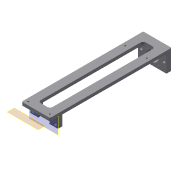
# Autodesk Inventor part: 02_Opentrons_Microscope_Base_v0
Saved by Autodesk Inventor 2019.4 (Build 234330000, 330)
## iProperties
Created: 2020-10-28
Part Number: 02_Opentrons_Microscope_Base_v0
Material: Generic
Document SubType Name: Modeling
Designer: diederichbenedict
Density: 1 g/cm^3
Appearance: Default
Author: diederichbenedict
Autodesk Inventor part; units mm, degrees
ref_plane "YZ Plane" through (0, 0, 0) normal (1, 0, 0) x (0, 1, 0)
ref_plane "XZ Plane" through (0, 0, 0) normal (0, 1, 0) x (-1, 0, 0)
ref_plane "XY Plane" through (0, 0, 0) normal (0, 0, 1) x (1, 0, 0)
ref_plane "Work Plane1" through (130.593, 54.6266, 280.0982) normal (0, 1, 0) x (1, 0, 0)
sketch "Sketch1" plane through (130.593, 54.6266, 280.0982) normal (0, 1, 0) x (1, 0, 0)
  line L0 (0, 36) -> (2, 38) projected
  line L1 (0, 27) -> (0, 36) projected
  line L2 (2, 25) -> (0, 27) projected
  line L3 (2, 25) -> (53, 25) projected
  line L4 (55, 27) -> (53, 25) projected
  line L5 (55, 27) -> (55, 36) projected
  line L6 (53, 38) -> (55, 36) projected
  line L7 (2, 38) -> (53, 38) projected
  circle A0 centre (6.5, 31.5) radius 2.5 construction
  circle A1 centre (48.5, 31.5) radius 2.5 construction
  line L8 (0, 224) -> (2, 226) projected
  line L9 (0, 215) -> (0, 224) projected
  line L10 (2, 213) -> (0, 215) projected
  line L11 (2, 213) -> (53, 213) projected
  line L12 (55, 215) -> (53, 213) projected
  line L13 (55, 215) -> (55, 224) projected
  line L14 (53, 226) -> (55, 224) projected
  line L15 (2, 226) -> (53, 226) projected
  circle A2 centre (6.5, 219.5) radius 2.5 construction
  circle A3 centre (48.5, 219.5) radius 2.5 construction
  line L16 (55, 25) -> (0, 25)
  line L17 (0, 25) -> (0, 261)
  line L18 (0, 261) -> (55, 261)
  line L19 (55, 261) -> (55, 25)
  line L20 (16, 261) -> (39, 261) projected
  circle A4 centre (48.5, 31.5) radius 1.45
  circle A5 centre (6.5, 31.5) radius 1.45
  circle A6 centre (48.5, 219.5) radius 1.45
  circle A7 centre (6.5, 219.5) radius 1.45
  point P0 (-130.593, 280.0982)
  dimension "d12" = 2.9
  dimension "d13" = 2.9
  dimension "d14" = 2.9
  dimension "d15" = 2.9
  constraints: 8 end point, 4 centre point, 3 coincident, 2 parallel, 2 point on line, 1 horizontal, 1 perpendicular
  measures "d12" diameter of A4
  measures "d13" diameter of A5
  measures "d14" diameter of A6
  measures "d15" diameter of A7
extrude "Extrusion1" add sketch "Sketch1" along normal blind 6
sketch "Sketch2" plane through (185.593, 54.6266, 19.0982) normal (0, 0, -1) x (-1, 0, 0)
  line L0 (46, 0) -> (46, 10) projected
  circle A0 centre (39, -26) radius 0.8 projected
  circle A1 centre (39, -3) radius 0.8 projected
  circle A2 centre (16, -26) radius 0.8 projected
  circle A3 centre (16, -3) radius 0.8 projected
  circle A4 centre (27.5, -14.5) radius 9.4 projected
  circle A5 centre (27.5, -14.5) radius 10.8 projected
  circle A6 centre (27.5, -14.5) radius 11.8
  circle A7 centre (5.5, -14.5) radius 3 projected
  circle A8 centre (49.5, -14.5) radius 3 projected
  circle A9 centre (5.5, -14.5) radius 3.1
  circle A10 centre (49.5, -14.5) radius 3.1
  line L1 (0, 0) -> (55, 0) projected
  line L2 (0, 0) -> (55, 0)
  line L3 (55, 0) -> (55, -32.5)
  line L4 (55, -32.5) -> (0, -32.5)
  line L5 (0, -32.5) -> (0, 0)
  point P0 (185.593, -54.6266)
  dimension "d2" = 1
  dimension "d3" = 6.2
  dimension "d4" = 6.2
  dimension "d5" = 18
  constraints: 8 end point, 3 centre point, 2 coincident, 2 parallel, 1 horizontal, 1 perpendicular
  measures "d2" radial gap between concentric circles of A5 A6
  measures "d3" diameter of A9
  measures "d4" diameter of A10
  measures "d5" distance from line of L4 A5.centre
extrude "Extrusion2" add sketch "Sketch2" against normal blind 10 contours L1 L3 L4 L5
ref_plane "Work Plane2" through (158.093, 40.1266, 239.5982) normal (0, 0, -1) x (1, 0, 0)
sketch "Sketch3" plane through (158.093, 40.1266, 239.5982) normal (0, 0, -1) x (1, 0, 0)
  circle A0 centre (-22, 0) radius 3 projected
  circle A1 centre (22, 0) radius 3 projected
  circle A2 centre (0, 0) radius 11.8 projected
  line L0 (27.5, -14.5) -> (27.5, -20.5) projected
  line L1 (-27.5, 18) -> (-27.5, -20.5) projected
  line L2 (27.5, -14.5) -> (-27.5, -14.5)
  line L3 (-27.5, -14.5) -> (-27.5, 5.5)
  line L4 (-27.5, 5.5) -> (27.5, 5.5)
  line L5 (27.5, 5.5) -> (27.5, -14.5)
  point P0 (-158.093, 40.1266)
  point P1 (10.4398, 5.5)
  point P2 (-10.4398, 5.5)
  dimension "d8" = 20
  constraints: 8 end point, 3 point on line, 2 parallel, 2 point on circle, 1 horizontal, 1 perpendicular
  measures "d8" distance of L2.end L3.end
extrude "Extrusion3" add sketch "Sketch3" along normal blind 10 contours A2 L4 L5 L2 L1
fillet "Fillet1" radius 2 9 edges at (185.593, 41.3766, 19.0982) (158.093, 54.6266, 29.0982) (185.593, 44.6266, 229.5982) (185.593, 44.6266, 239.5982) (130.593, 44.6266, 229.5982) (130.593, 44.6266, 239.5982) (130.593, 57.6266, 255.0982) (185.593, 57.6266, 255.0982) (130.593, 41.3766, 19.0982)
sketch "Sketch4" plane through (130.593, 60.6266, 280.0982) normal (0, 1, 0) x (1, 0, 0)
  arc A0 (2, 261) -> (0, 259) centre (2, 259) ccw construction
  line L0 (0, 259) -> (0, 27) construction
  arc A1 (0, 27) -> (2, 25) centre (2, 27) ccw construction
  line L1 (2, 25) -> (53, 25) construction
  arc A2 (53, 25) -> (55, 27) centre (53, 27) ccw construction
  line L2 (55, 27) -> (55, 259) construction
  arc A3 (55, 259) -> (53, 261) centre (53, 259) ccw construction
  line L3 (53, 261) -> (2, 261) construction
  circle A4 centre (6.5, 219.5) radius 1.45 projected
  circle A5 centre (48.5, 219.5) radius 1.45 projected
  circle A6 centre (6.5, 31.5) radius 1.45 projected
  circle A7 centre (48.5, 31.5) radius 1.45 projected
  line L4 (16, 46) -> (16, 240)
  line L5 (21, 245) -> (34, 245)
  line L6 (39, 240) -> (39, 46)
  line L7 (34, 41) -> (21, 41)
  arc A8 (16, 46) -> (21, 41) centre (21, 46) ccw
  arc A9 (34, 41) -> (39, 46) centre (34, 46) ccw
  arc A10 (39, 240) -> (34, 245) centre (34, 240) ccw
  arc A11 (21, 245) -> (16, 240) centre (21, 240) ccw
  point P0 (-130.593, 280.0982)
  dimension "d16" = 16
  dimension "d17" = 5
  constraints: 8 end point, 8 point on circle, 8 tangent, 4 centre point, 3 equal radius, 3 other
  measures "d16" distance between parallel lines of L0 L4
  measures "d17" radius of A8
extrude "Extrusion4" cut sketch "Sketch4" against normal through all contours L4 A11 L5 A10 L6 A9 L7 A8
sketch "Sketch5" plane through (130.593, 60.6266, 280.0982) normal (0, 1, 0) x (1, 0, 0)
  circle A0 centre (48.5, 219.5) radius 1.45 projected
  circle A1 centre (6.5, 219.5) radius 1.45 projected
  line L0 (0, 251) -> (55, 251) projected
  line L1 (0, 251) -> (55, 251) projected
  line L2 (0, 251) -> (55, 251) projected
  line L3 (16.8, 251) -> (15.2, 251) projected
  line L4 (16.8, 251) -> (15.2, 251) projected
  line L5 (39.8, 251) -> (38.2, 251) projected
  line L6 (39.8, 251) -> (38.2, 251) projected
  line L7 (52.6, 251) -> (46.4, 251) projected
  line L8 (8.6, 251) -> (2.4, 251) projected
  line L9 (39.3, 251) -> (15.7, 251) projected
  line L10 (53, 261) -> (2, 261) projected
  circle A2 centre (48.5, 256) radius 1.45
  circle A3 centre (6.5, 256) radius 1.45
  line L11 (55, 27) -> (55, 259) projected
  circle A4 centre (48.5, 219.5) radius 1.45
  circle A5 centre (6.5, 219.5) radius 1.45
  circle A6 centre (48.5, 183) radius 1.45
  circle A7 centre (6.5, 183) radius 1.45
  circle A8 centre (48.5, 146.5) radius 1.45
  circle A9 centre (6.5, 146.5) radius 1.45
  circle A10 centre (48.5, 110) radius 1.45
  circle A11 centre (6.5, 110) radius 1.45
  circle A12 centre (48.5, 73.5) radius 1.45
  circle A13 centre (6.5, 73.5) radius 1.45
  circle A14 centre (48.5, 37) radius 1.45
  circle A15 centre (6.5, 37) radius 1.45
  point P0 (-130.593, 280.0982)
  point P1 (53, 224.5)
  point P2 (55, 222.5)
  point P3 (2, 224.5)
  point P4 (53, 188)
  point P5 (55, 186)
  point P6 (2, 188)
  point P7 (53, 151.5)
  point P8 (55, 149.5)
  point P9 (2, 151.5)
  point P10 (53, 115)
  point P11 (55, 113)
  point P12 (2, 115)
  point P13 (53, 78.5)
  point P14 (55, 76.5)
  point P15 (2, 78.5)
  point P16 (53, 42)
  point P17 (55, 40)
  point P18 (2, 42)
  dimension "d20" = 2.9
  dimension "d21" = 2.9
  dimension "d22" = 5
  dimension "d23" = 5
  dimension "d24" = 36.5
  dimension "d27" = 36.5
  constraints: 14 centre point, 1 vertical, 42 other
  measures "d20" diameter of A2
  measures "d21" diameter of A3
  measures "d22" distance from line of A2.centre L10
  measures "d23" distance from line of L10 A3.centre
  measures "d24" distance of A0.centre A2.centre
  measures "d27" distance of L10.start point (53, 224.5)
extrude "Extrusion5" cut sketch "Sketch5" against normal blind 15 contours A2 | A3 | A6 | A7 | A8 | A9 | A10 | A11 | A12 | A13 | A14 | A15
body "Solid1"
